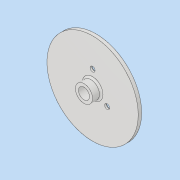
# Autodesk Inventor part: SmallSpoolEndFore
Saved by Autodesk Inventor 2017 (Build 210142000, 142)
## iProperties
Created: 2018-04-03
Part Number: SmallSpoolEndFore
Material: ABS Plastic
Document SubType Name: Modeling
Designer: Derek Wider
Density: 1.06 g/cm^3
Appearance: Smooth - White
Author: Derek Wider
Autodesk Inventor part; units mm, degrees
ref_plane "YZ Plane" through (0, 0, 0) normal (1, 0, 0) x (0, 1, 0)
ref_plane "XZ Plane" through (0, 0, 0) normal (0, 1, 0) x (-1, 0, 0)
ref_plane "XY Plane" through (0, 0, 0) normal (0, 0, 1) x (1, 0, 0)
sketch "Sketch1" plane through (0, 0, 0) normal (0, 0, 1) x (1, 0, 0)
  circle A0 centre (0, 0) radius 33.655
  dimension "d0" = 67.31
  constraints: 1 centre point, 1 coincident
  measures "d0" diameter of A0
extrude "Extrusion1" add sketch "Sketch1" along normal blind 2.54
sketch "Sketch2" plane through (0, 0, 0) normal (0, 0, -1) x (-1, 0, 0)
  circle A0 centre (0, 12.3825) radius 1.8415
  point P0 (0, 0)
  dimension "d3" = 3.683
  dimension "d4" = 12.3825
  constraints: 1 centre point
  measures "d3" diameter of A0
  measures "d4" distance of point (0, 0) A0.centre
extrude "Extrusion2" cut sketch "Sketch2" against normal through all
chamfer "Chamfer1" distance 1.27 angle 45 1 edges at (1.8415, 12.3825, 0)
pattern_circular "Circular Pattern1" count 3 over 360 about axis through (0, 0, 0) along (0, 0, 1) of "Extrusion2", "Chamfer1"
sketch "Sketch3" plane through (0, 0, 2.54) normal (0, 0, 1) x (1, 0, 0)
  circle A0 centre (0, 0) radius 6.35
  circle A1 centre (0, 0) radius 3.4925
  circle A2 centre (0, 0) radius 4.064
  dimension "d13" = 12.7
  dimension "d14" = 6.985
  dimension "d15" = 8.128
  constraints: 3 centre point, 3 coincident
  measures "d13" diameter of A0
  measures "d14" diameter of A1
  measures "d15" diameter of A2
extrude "Extrusion3" add sketch "Sketch3" along normal blind 6.35 contours A0
extrude "Extrusion4" cut sketch "Sketch3" against normal through all contours A1
fillet "Fillet1" radius 1.27 1 edges at (-6.35, 0, 2.54)
body "Solid1"
